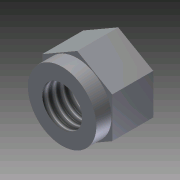
# Autodesk Inventor part: Big Nut 1764
Saved by Autodesk Inventor 2011 (Build 150239000, 239)
## iProperties
Created: 2010-02-11
Part Number: Big Nut 1764
Document SubType Name: Modeling
Designer: jrobinson
Density: 1 g/cm^3
Author: jrobinson
Autodesk Inventor part; units mm, degrees
ref_plane "YZ Plane" through (0, 0, 0) normal (1, 0, 0) x (0, 1, 0)
ref_plane "XZ Plane" through (0, 0, 0) normal (0, 1, 0) x (-1, 0, 0)
ref_plane "XY Plane" through (0, 0, 0) normal (0, 0, 1) x (1, 0, 0)
sketch "Sketch1" plane through (0, 0, 0) normal (0, 0, 1) x (1, 0, 0)
  line L0 (-12.2264, 9.7457) -> (-5.1779, 13.8152)
  line L1 (-5.1779, 13.8152) -> (1.8706, 9.7457)
  line L2 (1.8706, 9.7457) -> (1.8706, 1.6068)
  line L3 (1.8706, 1.6068) -> (-5.1779, -2.4626)
  line L4 (-5.1779, -2.4626) -> (-12.2264, 1.6068)
  line L5 (-12.2264, 1.6068) -> (-12.2264, 9.7457)
  point P0 (0, 0)
  point P1 (-5.1779, 5.6763)
  dimension "d0" = 14.097
  constraints: 12 end point, 1 vertical, 13 other
  measures "d0" distance between parallel lines of L5 L2
extrude "Extrusion1" add sketch "Sketch1" along normal blind 8.255
sketch "Sketch2" plane through (0, 0, 8.255) normal (0, 0, 1) x (1, 0, 0)
  circle A0 centre (-5.1779, 5.6763) radius 6.8961
  point P0 (0, 0)
  dimension "d3" = 13.7922
  constraints: 1 centre point
  measures "d3" diameter of A0
extrude "Extrusion2" add sketch "Sketch2" along normal blind 3.048
sketch "Sketch3" plane through (-5.1779, 5.6763, 11.303) normal (0, 0, 1) x (1, 0, 0)
  circle A0 centre (0, 0) radius 6.8961 projected
  circle A1 centre (0, 0) radius 4.0005
  point P0 (5.1779, -5.6763)
  dimension "d6" = 8.001
  constraints: 1 centre point, 1 coincident
  measures "d6" diameter of A1
extrude "Extrusion3" cut sketch "Sketch3" against normal through all contours A1
thread "Thread1" size "3/8-16 UNC" class "2B" standard "ANSI Unified Screw Threads" full length
body "Solid1"
